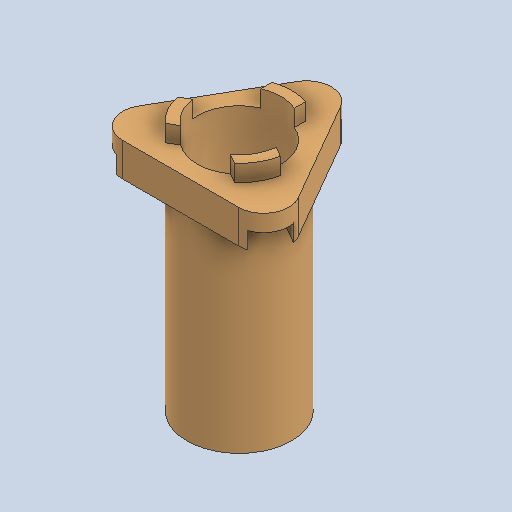
# Autodesk Inventor part: Suporte Contato
Saved by Autodesk Inventor 2022.2 (Build 262287000, 287)
## iProperties
Created: 2021-01-22
Part Number: Suporte Contato
Material: Genérico
Document SubType Name: Modeling
Designer: João
Density: 1 g/cm^3
Appearance: Padrão
Mass: 0.00158181 g
Surface Area: 0.260234 cm^2
Volume: 0.00158181 cm^3
Author: João
Autodesk Inventor part; units mm, degrees
ref_plane "YZ Plane" through (0, 0, 0) normal (1, 0, 0) x (0, 1, 0)
ref_plane "XZ Plane" through (0, 0, 0) normal (0, 1, 0) x (-1, 0, 0)
ref_plane "XY Plane" through (0, 0, 0) normal (0, 0, 1) x (1, 0, 0)
sketch "Esboço1" plane through (0, 0, 0) normal (0, 1, 0) x (-1, 0, 0)
  circle A0 centre (0, 0) radius 0.625
  circle A1 centre (0, 0) radius 0.5
  dimension "d0" = 1.25
  dimension "d1" = 1
  constraints: 2 centre point, 2 coincident
  measures "d0" diameter of A0
  measures "d1" diameter of A1
extrude "Extrusão1" add sketch "Esboço1" against normal blind 2.8
sketch "Esboço2" plane through (0, 0, 0) normal (0, 1, 0) x (1, 0, 0)
  line L0 (0, 0) -> (0, 1.4)
  line L1 (0, 0) -> (0, -1.4)
  line L2 (0, 0) -> (-1.2124, -0.7)
  line L3 (0, 0) -> (1.2124, -0.7)
  line L4 (0.2598, 0.95) -> (0.9526, -0.25)
  line L5 (-0.9526, -0.25) -> (-0.2598, 0.95)
  line L6 (-0.6928, -0.7) -> (0.6928, -0.7)
  arc A0 (-0.9526, -0.25) -> (-0.6928, -0.7) centre (-0.6928, -0.4) ccw
  arc A1 (0.6928, -0.7) -> (0.9526, -0.25) centre (0.6928, -0.4) ccw
  arc A2 (0.2598, 0.95) -> (-0.2598, 0.95) centre (0, 0.8) ccw
  circle A3 centre (0, 0) radius 0.625 projected
  circle A4 centre (0, 0) radius 0.5 projected
  dimension "d5" = 1.4
  dimension "d6" = 1.4
  dimension "d9" = 360
  dimension "d11" = 0.3
  constraints: 14 end point, 6 point on circle, 6 point on line, 6 tangent, 3 centre point, 2 coincident, 2 equal radius, 2 vertical, 1 horizontal, 8 other
  measures "d5" distance of L0.start L0.end
  measures "d6" distance of L0.start L1.end
  measures "d11" radius of A0
extrude "Extrusão2" add sketch "Esboço2" against normal blind 0.4 contours A3 L2 A0 L5 A2 L0 | L0 A2 L4 A1 L3 A3 | A3 L3 A1 L6 L1 | L1 L6 A0 L2 A3
sketch "Esboço3" plane through (0, -0.4, 0) normal (0, -1, 0) x (1, 0, 0)
  line L0 (0.2, 0) -> (-0.2, 0)
  line L1 (-0.2, 0) -> (-0.2, -1.1589)
  line L2 (-0.2, -1.1589) -> (0.2, -1.1589)
  line L3 (0.2, -1.1589) -> (0.2, 0)
  line L4 (-0.1, 0.1732) -> (0.1, -0.1732)
  line L5 (0.1, -0.1732) -> (1.1036, 0.4062)
  line L6 (1.1036, 0.4062) -> (0.9036, 0.7526)
  line L7 (0.9036, 0.7526) -> (-0.1, 0.1732)
  line L8 (-0.1, -0.1732) -> (0.1, 0.1732)
  line L9 (0.1, 0.1732) -> (-0.9036, 0.7526)
  line L10 (-0.9036, 0.7526) -> (-1.1036, 0.4062)
  line L11 (-1.1036, 0.4062) -> (-0.1, -0.1732)
  arc A0 (0.9526, 0.25) -> (0.6928, 0.7) centre (0.6928, 0.4) ccw projected
  line L12 (0.6928, 0.7) -> (-0.6928, 0.7) projected
  arc A1 (-0.6928, 0.7) -> (-0.9526, 0.25) centre (-0.6928, 0.4) ccw projected
  line L13 (-0.9526, 0.25) -> (-0.2598, -0.95) projected
  arc A2 (-0.2598, -0.95) -> (0.2598, -0.95) centre (0, -0.8) ccw projected
  line L14 (0.2598, -0.95) -> (0.9526, 0.25) projected
  circle A3 centre (0, 0) radius 0.625 projected
  circle A4 centre (0, 0) radius 0.625 projected
  circle A5 centre (0, 0) radius 0.5 projected
  circle A6 centre (0, 0) radius 0.625 projected
  circle A7 centre (0, 0) radius 0.675
  point P0 (0.2, -0.6447)
  point P1 (0.6583, 0.1491)
  point P2 (0.9865, 0.3386)
  point P3 (0.7865, 0.685)
  point P4 (0.4583, 0.4956)
  point P5 (-0.4583, 0.4956)
  point P6 (-0.7865, 0.685)
  point P7 (-0.9865, 0.3386)
  point P8 (-0.6583, 0.1491)
  point P9 (-0.2, -0.6447)
  point P10 (-0.2, -1.0236)
  point P11 (0.2, -1.0236)
  dimension "d14" = 0.4
  dimension "d17" = 360
  dimension "d20" = 1.35
  constraints: 24 end point, 3 coincident, 2 parallel, 1 centre point, 1 horizontal, 1 perpendicular, 26 other
  measures "d14" distance of L2.end L1.end
  measures "d20" diameter of A7
extrude "Extrusão3" cut sketch "Esboço3" against normal blind 0.2 contours A3 L5 A7 L3 | L3 A7 L1 A3 | A3 L7 A7 L5 | L3 A2 L1 A7 | L1 A7 L11 A3 | A7 L7 A0 L5 | A3 L9 A7 L7 | L11 A7 L9 A3 | L11 A1 L9 A7
sketch "Esboço4" plane through (0, 0, 0) normal (0, 1, 0) x (1, 0, 0)
  circle A0 centre (0, 0) radius 0.6
  line L0 (0.9865, -0.3386) -> (0.6583, -0.1491) projected
  arc A1 (0.7865, -0.685) -> (0.9865, -0.3386) centre (0.6928, -0.4) ccw projected
  line L1 (0.4583, -0.4956) -> (0.7865, -0.685) projected
  arc A2 (-0.4583, -0.4956) -> (0.4583, -0.4956) centre (0, 0) ccw projected
  line L2 (-0.7865, -0.685) -> (-0.4583, -0.4956) projected
  arc A3 (-0.9865, -0.3386) -> (-0.7865, -0.685) centre (-0.6928, -0.4) ccw projected
  line L3 (-0.6583, -0.1491) -> (-0.9865, -0.3386) projected
  arc A4 (-0.2, 0.6447) -> (-0.6583, -0.1491) centre (0, 0) ccw projected
  line L4 (-0.2, 1.0236) -> (-0.2, 0.6447) projected
  arc A5 (0.2, 1.0236) -> (-0.2, 1.0236) centre (0, 0.8) ccw projected
  line L5 (0.2, 0.6447) -> (0.2, 1.0236) projected
  arc A6 (0.6583, -0.1491) -> (0.2, 0.6447) centre (0, 0) ccw projected
  circle A7 centre (0, 0) radius 0.625 projected
  line L6 (0.9036, -0.7526) -> (-0.1, -0.1732) projected
  line L7 (0.1, 0.1732) -> (1.1036, -0.4062) projected
  line L8 (0.1, -0.1732) -> (-0.9036, -0.7526) projected
  line L9 (-1.1036, -0.4062) -> (-0.1, 0.1732) projected
  line L10 (-0.2, 0) -> (-0.2, 1.1589) projected
  line L11 (0.2, 1.1589) -> (0.2, 0) projected
  circle A8 centre (0, 0) radius 0.5
  point P0 (-0.2, 0.4583)
  point P1 (0.2, 0.4583)
  point P2 (0.2, 0.5921)
  point P3 (-0.2, 0.5921)
  point P4 (0.4969, -0.0559)
  point P5 (0.2969, -0.4023)
  point P6 (0.4128, -0.4693)
  point P7 (0.6128, -0.1229)
  point P8 (-0.2969, -0.4023)
  point P9 (-0.4969, -0.0559)
  point P10 (-0.6128, -0.1229)
  point P11 (-0.4128, -0.4693)
  dimension "d23" = 1.2
  dimension "d24" = 1
  constraints: 2 centre point, 2 coincident
  measures "d23" diameter of A0
  measures "d24" diameter of A8
extrude "Extrusão4" add sketch "Esboço4" along normal blind 0.2 contours L11 A8 L10 A0 | A0 L10 A7 L11 | L7 A7 L6 A0 | A0 L6 A8 L7 | L9 A8 L8 A0 | A0 L8 A7 L9
